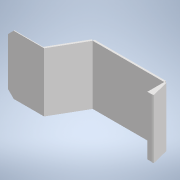
# Autodesk Inventor part: ДИ 00,00,01
Saved by Autodesk Inventor 2021.2 (Build 252289000, 289)
## iProperties
Created: 2021-10-11
Part Number: ДИ 00,00,01
Material: Типовые
Document SubType Name: Modeling
Designer: Surflay
Density: 1 g/cm^3
Appearance: По умолчанию
Author: Surflay
Autodesk Inventor part; units mm, degrees
sketch "Эскиз1" plane through (0, 0, 0) normal (0, 0, 1) x (1, 0, 0)
  line L0 (0, 0) -> (-247, 0)
  line L1 (-247, 0) -> (-247, -204)
  line L2 (-247, -204) -> (0, -204)
  line L3 (0, -204) -> (0, 0)
  dimension "d0" = 247
  dimension "d1" = 204
  constraints: 8 end point, 2 parallel, 1 horizontal, 1 perpendicular
  measures "d0" distance of L2.end L1.end
  measures "d1" distance of L1.end L0.end
extrude "Выдавливание1" add sketch "Эскиз1" along normal blind 6.4
ref_plane "РабПлоскость1" through (-247, 0, 6.4) normal (-0.8660254, 0, -0.5) x (0, -1, 0)
sketch "Эскиз2" plane through (-247, 0, 6.4) normal (-0.8660254, 0, -0.5) x (0, -1, 0)
  line L0 (0, 0) -> (204, 0) projected
  line L1 (204, 0) -> (0, 0)
  line L2 (0, 0) -> (0, 123)
  line L3 (0, 123) -> (204, 123)
  line L4 (204, 123) -> (204, 0)
  point P0 (0, -129.0426)
  dimension "d5" = 123
  constraints: 8 end point, 2 parallel, 1 horizontal, 1 perpendicular
  measures "d5" distance of L0.start L2.end
extrude "Выдавливание2" add sketch "Эскиз2" along normal blind 6.4
ref_plane "РабПлоскость2" through (0, -204, 6.4) normal (0.9702957, 0, -0.2419219) x (0, 1, 0)
sketch "Эскиз3" plane through (0, -204, 6.4) normal (0.9702957, 0, -0.2419219) x (0, 1, 0)
  line L0 (204, 0) -> (204, -59.7547) projected
  line L1 (204, 0) -> (0, 0)
  line L2 (0, 0) -> (0, 60)
  line L3 (0, 60) -> (204, 60)
  line L4 (204, 60) -> (204, 0)
  point P0 (204, -6.2099)
  dimension "d9" = 60
  constraints: 8 end point, 2 parallel, 1 coincident, 1 horizontal, 1 perpendicular
  measures "d9" distance of L1.end L2.end
extrude "Выдавливание3" add sketch "Эскиз3" along normal blind 6.4
ref_plane "РабПлоскость3" through (-308.5, -204, 112.9211) normal (0, 0, -1) x (0, 1, 0)
sketch "Эскиз4" plane through (-308.5, -204, 112.9211) normal (0, 0, -1) x (0, 1, 0)
  line L0 (0, 0) -> (204, 0) projected
  line L1 (204, 0) -> (0, 0)
  line L2 (0, 0) -> (0, -125)
  line L3 (0, -125) -> (204, -125)
  line L4 (204, -125) -> (204, 0)
  point P0 (204, 308.5)
  dimension "d13" = 125
  constraints: 8 end point, 2 parallel, 1 horizontal, 1 perpendicular
  measures "d13" distance of L0.start L2.end
extrude "Выдавливание4" add sketch "Эскиз4" along normal blind 2.5
chamfer "Фаска1" distance 20 angle 45 2 edges at (-433.5, -204, 111.6711) (-433.5, 0, 111.6711)
sketch "Эскиз5" plane through (0, -204, 0) normal (1, 0, 0) x (0, 0, -1)
  line L0 (-6.4, 0) -> (-6.4, 204) projected
  line L1 (-6.4, 204) -> (-64.6177, 204) projected
  line L2 (-6.4, 1.5695) -> (-64.6177, 1.5695)
  line L3 (-64.6177, 1.5695) -> (-64.6177, 204)
  line L4 (-64.6177, 204) -> (-6.4, 204)
  line L5 (-6.4, 204) -> (-6.4, 1.5695)
  point P0 (0, 204)
  constraints: 8 end point, 2 parallel, 1 horizontal, 1 perpendicular, 1 point on line
extrude "Выдавливание5" add sketch "Эскиз5" against normal up to surface surface through (7.2577, -102, 35.5089) normal (0.9702957, 0, -0.2419219)
